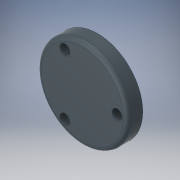
# Autodesk Inventor part: AA014
Saved by Autodesk Inventor 2017 SP1 (Build 210196100, 196)
## iProperties
Created: 2017-09-29
Part Number: AA014
Material: ABS Plastic
Document SubType Name: Modeling
Designer: Zach
Density: 1.06 g/cm^3
Appearance: CR Dark Blue
Author: Zach
Autodesk Inventor part; units mm, degrees
ref_plane "YZ Plane" through (0, 0, 0) normal (1, 0, 0) x (0, 1, 0)
ref_plane "XZ Plane" through (0, 0, 0) normal (0, 1, 0) x (-1, 0, 0)
ref_plane "XY Plane" through (0, 0, 0) normal (0, 0, 1) x (1, 0, 0)
sketch "Sketch1" plane through (0, 0, 0) normal (0, 0, 1) x (1, 0, 0)
  circle A0 centre (0, 0) radius 22
  circle A1 centre (17, 0) radius 2.5
  circle A2 centre (-8.5, 14.7224) radius 2.5
  circle A3 centre (-8.5, -14.7224) radius 2.5
  dimension "d0" = 44
  dimension "d1" = 5
  dimension "d2" = 17
  dimension "d5" = 360
  constraints: 4 centre point, 1 coincident, 1 horizontal alignment, 7 other
  measures "d0" diameter of A0
  measures "d1" diameter of A1
  measures "d2" distance of A1.centre point (0, 0)
extrude "Extrusion1" add sketch "Sketch1" along normal blind 7.5
fillet "Fillet1" radius 2 1 edges at (-22, 0, 7.5)
sketch "Sketch2" plane through (0, 0, 0) normal (0, 0, -1) x (-1, 0, 0)
  circle A0 centre (0, 0) radius 4.15
  dimension "d10" = 8.3
  constraints: 1 centre point, 1 coincident
  measures "d10" diameter of A0
extrude "Extrusion2" cut sketch "Sketch2" against normal blind 5
body "Solid1"
